# Autodesk Inventor part: 同步皮带轮1
Saved by Autodesk Inventor 2015 (Build 190159000, 159)
## iProperties
Created: 2017-05-28
Part Number: 同步皮带轮1
Material: Steel
Document SubType Name: Modeling
Designer: Administrator
Density: 1 g/cm^3
Appearance: Steel
CustomPartVersion: 1
Author: Administrator
Autodesk Inventor part; units mm, degrees
ref_plane "YZ Plane" through (0, 0, 0) normal (1, 0, 0) x (0, 1, 0)
ref_plane "XZ Plane" through (0, 0, 0) normal (0, 1, 0) x (-1, 0, 0)
ref_plane "XY Plane" through (0, 0, 0) normal (0, 0, 1) x (1, 0, 0)
sketch "皮带轮草图" plane through (0, 0, 0) normal (0, 0, 1) x (1, 0, 0)
  circle A0 centre (0, 0) radius 24.2552 construction
  circle A1 centre (0, 0) radius 23.5694
  circle A2 centre (0, 0) radius 20.5214
  line L0 (-3.129, 23.3608) -> (-2.0955, 20.5214)
  line L1 (-2.0955, 20.5214) -> (2.0955, 20.5214)
  line L2 (2.0955, 20.5214) -> (3.129, 23.3608)
  line L3 (0, 0) -> (0, 23.5694) construction
  point P0 (0, 20.5214)
  dimension "d0" = 48.5104
  dimension "d1" = 0.6858
  dimension "d2" = 3.048
  dimension "d3" = 40
  dimension "d4" = 4.191
  constraints: 8 end point, 3 coincident, 3 point on circle, 2 centre point, 1 horizontal, 1 midpoint, 1 point on line, 1 vertical, 1 vertical alignment, 3 other
  measures "d0" diameter of A0
  measures "d1" radial gap between concentric circles of A0 A1
  measures "d3" angle of L2 L0
  measures "d4" distance of L0.end L1.end
extrude "基础实体" add sketch "皮带轮草图" along normal mid plane 20 contours A2 | A1 L0 L1 L2 | L2 L1 L0 A1
extrude "齿" cut sketch "皮带轮草图" along normal through all both and the other way through all contours L2 L1 L0 A1 picked at (-1.0471, 21.5297)
fillet "Fillet" radius 1.6002 2 edges at (2.0955, 20.5214, 0) (-2.0955, 20.5214, 0)
fillet "Fillet" radius 1.6002 4 edges at (-3.129, 23.3608, 5) (-3.129, 23.3608, -5) (3.129, 23.3608, 5) (3.129, 23.3608, -5)
pattern_circular "Teeth" count 12 over 360 about axis through (0, 0, -10) along (0, 0, 1) of "齿", "Fillet"
pulley flange "左侧凸缘" diameter 47.1388 height 1.5 thickness 1.5 bend angle 10 centre (0, 0, -10) toward (0, 0, -1)
pulley flange "右侧凸缘" diameter 47.1388 height 1.5 thickness 1.5 bend angle 10 centre (0, 0, 10) toward (0, 0, 1)
equation "\"d1\" = da_a"
equation "\"d2\" = da_hg"
equation "\"d3\" = 2 * da_fi"
equation "\"d4\" = da_bw"
equation "\"d5\" = da_bf"
equation "\"d7\" = da_bf"
equation "\"d9\" = da_rb"
equation "\"d10\" = da_rt"
equation "\"da_pb\" = 12.7"
equation "\"da_fi\" = 20deg"
equation "\"da_hg\" = 3.048"
equation "\"da_bw\" = 4.191"
equation "\"da_rb\" = 1.6002"
equation "\"da_rt\" = 1.6002"
equation "\"da_a\" = 0.6858"
equation "\"da_bf\" = 20"
equation "\"da_wf\" = 1.5"
equation "\"da_hf\" = 1.5"
body "Solid1"
